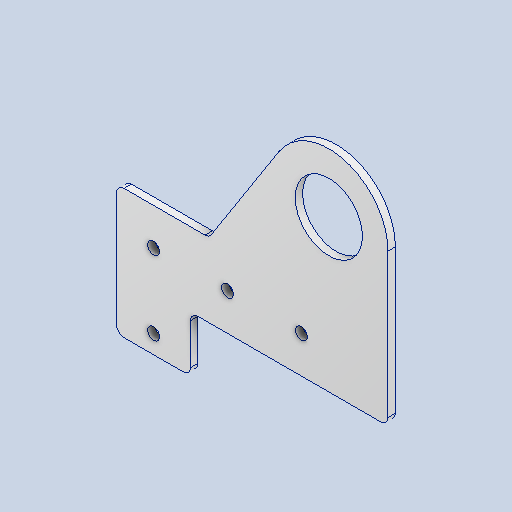
# Autodesk Inventor part: dribl-v3-Plate-1
Saved by Autodesk Inventor 2025.2 (Build 292293000, 293)
## iProperties
Created: 2025-04-04
Part Number: dribl-v3-Plate-1
Material: アルミニウム 6061
Document SubType Name: Modeling
Designer: haruy
Density: 2.7 g/cm^3
Appearance: アルミニウム - フラット
Author: haruy
Autodesk Inventor part; units mm, degrees
ref_plane "YZ Plane" through (0, 0, 0) normal (1, 0, 0) x (0, 1, 0)
ref_plane "XZ Plane" through (0, 0, 0) normal (0, 1, 0) x (-1, 0, 0)
ref_plane "XY Plane" through (0, 0, 0) normal (0, 0, 1) x (1, 0, 0)
derived "dribl-v3-Sketch-Base.ipt"
sketch "スケッチ5" plane through (-180, -184.3334, -303) normal (0, 0, 1) x (1, 0, 0)
  circle A0 centre (37.42, 41) radius 16 projected
  line L0 (0, -248) -> (0, 1189.5) projected
  line L1 (560, 20) -> (0, 20) projected
  circle A1 centre (10, 10) radius 1.6 projected
  circle A2 centre (30, 10) radius 1.6 projected
  line L2 (0, 0) -> (560, 0) projected
  line L3 (280, 20) -> (280, 0) projected
  circle A3 centre (522.58, 41) radius 16 projected
  circle A4 centre (530, 10) radius 1.6 projected
  circle A5 centre (550, 10) radius 1.6 projected
  circle A6 centre (-10, 10) radius 1.6 projected
  circle A7 centre (-10, -10) radius 1.6 projected
  line L4 (-20, 1189.5) -> (-20, -248) projected
  circle A8 centre (570, 10) radius 1.6 projected
  circle A9 centre (570, -10) radius 1.6 projected
  circle A10 centre (37.42, 41) radius 16
  circle A11 centre (37.42, 41) radius 9.1
  line L5 (0, 20) -> (5, 20)
  line L6 (5, 20) -> (5, 63.0652)
  line L7 (5, 63.0652) -> (0, 63.0652)
  line L8 (0, 63.0652) -> (0, 20)
  line L9 (23.9403, 49.6196) -> (5, 20)
  line L10 (0, 20) -> (-20, 20)
  line L11 (-20, -15) -> (0, -15)
  line L12 (53.42, 41) -> (53.42, 0)
  point P0 (180, 184.3334)
  point P1 (53.42, 41)
  point P2 (23.9403, 49.6196)
  dimension "d1" = 32
  dimension "d2" = 18.2
  dimension "d3" = 5
  dimension "d4" = 5
  constraints: 16 end point, 4 perpendicular, 4 point on line, 2 centre point, 2 coincident, 2 parallel, 2 point on circle, 2 tangent, 1 horizontal
  measures "d1" diameter of A10
  measures "d2" diameter of A11
  measures "d3" distance of L7.end L6.end
  measures "d4" distance from line of L11 A7.centre
extrude "押し出し1" add sketch "スケッチ5" against normal blind 2 contours A0 | L12 L1 L9 A0 | L12 L2 L0 L1 | L0 L11 L4 L10
fillet "フィレット1" radius 2 6 edges at (-126.58, -184.3334, -304) (-180, -184.3334, -304) (-180, -199.3334, -304) (-200, -199.3334, -304) (-200, -164.3334, -304) (-175, -164.3334, -304)
